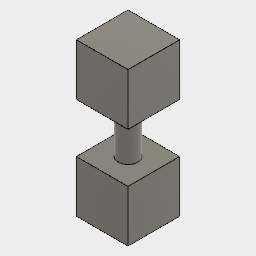
Гантеля1 v1 (Autodesk Fusion 360 design; units mm, degrees)
Autodesk Fusion 360 part; units mm, degrees
cylinder "CylinderPrimitive1" add diameter 40 height 100 placed x (1, 0, 0) y (0, 0, -1) z (0, 1, 0) at (0, 0, 0)
box "BoxPrimitive1" add length 100 width 100 height 105 placed x (0, 0, -1) y (-1, 0, 0) z (0, 1, 0) at (50, 100, 50)
extrude "Extrude1" add 1 faces at (16.6667, 135, 50) along direction (0, 0, 1) blind 2.5
extrude "Extrude2" add 1 faces at (16.6667, 135, -50) along direction (0, 0, -1) blind 2.5
box "BoxPrimitive2" add length 100 width 100 height 105 placed x (0, 0, -1) y (1, 0, 0) z (0, -1, 0) at (-50, 0, 50)
extrude "Extrude3" add 1 faces at (-16.6667, -35, -50) along direction (0, 0, -1) blind 2.5
extrude "Extrude4" add 1 faces at (-16.6667, -35, 50) along direction (0, 0, 1) blind 2.5
extrude "Extrude5" add 1 faces at (-50, -35, -17.5) along direction (-1, 0, 0) blind 2.5
extrude "Extrude6" add 1 faces at (-50, 170, -17.5) along direction (-1, 0, 0) blind 2.5
extrude "Extrude7" add 1 faces at (50, 170, -17.5) along direction (1, 0, 0) blind 2.5
extrude "Extrude8" add 1 faces at (50, -35, -17.5) along direction (1, 0, 0) blind 2.5
extrude "Extrude9" add 1 faces at (-52.5, -35, -17.5) along direction (-1, 0, 0) blind 2.5
extrude "Extrude10" cut 1 faces at (52.5, -35, -17.5) along direction (-1, 0, 0) blind 2.5
extrude "Extrude11" cut 1 faces at (15, -105, -17.5) along direction (0, 1, 0) blind 2.5
extrude "Extrude12" add 1 faces at (50, -68.3333, -17.5) along direction (1, 0, 0) blind 2.5
extrude "Extrude13" cut 1 faces at (-55, -68.3333, -17.5) along direction (1, 0, 0) blind 2.5
extrude "Extrude14" add 1 faces at (-17.5, -102.5, -17.5) along direction (0, -1, 0) blind 2.5
box "BoxPrimitive3" cut length 97 width 97 height -101 placed x (0, 0, -1) y (-1, 0, 0) z (0, 1, 0) at (48.5, 205, 48.5)
box "BoxPrimitive4" add length 97 width 97 height -4 placed x (0, 0, 1) y (1, 0, 0) z (0, 1, 0) at (-48.5, 205, -48.5)
box "BoxPrimitive5" cut length 97 width 97 height -101 placed x (0, 0, 1) y (-1, 0, 0) z (0, -1, 0) at (48.5, -105, -48.5)
box "BoxPrimitive6" add length 97 width 97 height -4 placed x (0, 0, 1) y (-1, 0, 0) z (0, -1, 0) at (48.5, -105, -48.5)
box "BoxPrimitive7" cut length 69 width 29 height -4 placed x (0, 1, 0) y (1, 0, 0) z (0, 0, -1) at (-14.5, -87, -52.5)
cylinder "CylinderPrimitive2" cut diameter 11 height -4 placed x (0, 1, 0) y (1, 0, 0) z (0, 0, -1) at (28, -25, -52.5)
